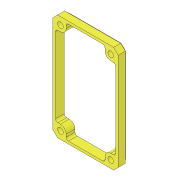
# Autodesk Inventor part: COXA_YAW_ROLL_ADPT_SPACER_2
Saved by Autodesk Inventor 2019.4 (Build 234330000, 330)
## iProperties
Created: 2019-11-06
Part Number: COXA_YAW_ROLL_ADPT_SPACER_2
Material: 一般
Document SubType Name: Modeling
Designer: y6tada
Density: 1 g/cm^3
Appearance: 滑らか - 黄
Author: y6tada
Autodesk Inventor part; units mm, degrees
ref_plane "YZ Plane" through (0, 0, 0) normal (1, 0, 0) x (0, 1, 0)
ref_plane "XZ Plane" through (0, 0, 0) normal (0, 1, 0) x (-1, 0, 0)
ref_plane "XY Plane" through (0, 0, 0) normal (0, 0, 1) x (1, 0, 0)
sketch "スケッチ1" plane through (0, 0, 0) normal (0, 0, 1) x (1, 0, 0)
  line L0 (-12.25, 11.25) -> (12.25, 11.25)
  line L1 (14.25, 9.25) -> (14.25, -33.25)
  line L2 (12.25, -35.25) -> (-12.25, -35.25)
  line L3 (-14.25, -33.25) -> (-14.25, 9.25)
  line L4 (-12.25, 11.25) -> (-14.25, 9.25)
  line L5 (12.25, 11.25) -> (14.25, 9.25)
  line L6 (14.25, -33.25) -> (12.25, -35.25)
  line L7 (-12.25, -35.25) -> (-14.25, -33.25)
  line L8 (0, 0) -> (-26.5626, 0) construction
  line L9 (0, 0) -> (0, 27.9433) construction
  line L10 (-11, 8) -> (11, 8) construction
  line L11 (11, 8) -> (11, -32) construction
  line L12 (11, -32) -> (-11, -32) construction
  line L13 (-11, -32) -> (-11, 8) construction
  line L14 (-13.15, -28.5) -> (-13.15, 4.5)
  line L15 (-7.5, 10.15) -> (7.5, 10.15)
  line L16 (13.15, 4.5) -> (13.15, -28.5)
  line L17 (7.5, -34.15) -> (-7.5, -34.15)
  line L18 (8.5, 8) -> (8.5, 9.15)
  line L19 (11, 5.5) -> (12.15, 5.5)
  arc A0 (8.5, 8) -> (11, 5.5) centre (11, 8) ccw
  line L20 (12.15, -29.5) -> (11, -29.5)
  line L21 (8.5, -32) -> (8.5, -33.15)
  arc A1 (11, -29.5) -> (8.5, -32) centre (11, -32) ccw
  line L22 (-8.5, 8) -> (-8.5, 9.15)
  line L23 (-11, 5.5) -> (-12.15, 5.5)
  arc A2 (-11, 5.5) -> (-8.5, 8) centre (-11, 8) ccw
  line L24 (-12.15, -29.5) -> (-11, -29.5)
  line L25 (-8.5, -32) -> (-8.5, -33.15)
  arc A3 (-8.5, -32) -> (-11, -29.5) centre (-11, -32) ccw
  arc A4 (8.5, 9.15) -> (7.5, 10.15) centre (7.5, 9.15) ccw
  arc A5 (13.15, 4.5) -> (12.15, 5.5) centre (12.15, 4.5) ccw
  arc A6 (12.15, -29.5) -> (13.15, -28.5) centre (12.15, -28.5) ccw
  arc A7 (7.5, -34.15) -> (8.5, -33.15) centre (7.5, -33.15) ccw
  arc A8 (-8.5, -33.15) -> (-7.5, -34.15) centre (-7.5, -33.15) ccw
  arc A9 (-13.15, -28.5) -> (-12.15, -29.5) centre (-12.15, -28.5) ccw
  arc A10 (-12.15, 5.5) -> (-13.15, 4.5) centre (-12.15, 4.5) ccw
  arc A11 (-7.5, 10.15) -> (-8.5, 9.15) centre (-7.5, 9.15) ccw
  point P0 (-14.25, 11.25)
  point P1 (14.25, -35.25)
  point P2 (14.25, 11.25)
  point P3 (-14.25, -35.25)
  point P4 (8.5, 10.15)
  point P5 (13.15, 5.5)
  point P6 (13.15, -29.5)
  point P7 (8.5, -34.15)
  point P8 (-8.5, 10.15)
  point P9 (-13.15, 5.5)
  point P10 (-13.15, -29.5)
  point P11 (-8.5, -34.15)
  dimension "d0" = 2
  dimension "d1" = 2
  dimension "d2" = 2
  dimension "d3" = 2
  dimension "d4" = 2
  dimension "d5" = 2
  dimension "d6" = 2
  dimension "d7" = 2
  dimension "d8" = 28.5
  dimension "d9" = 11.25
  dimension "d10" = 46.5
  dimension "d11" = 8
  dimension "d12" = 22
  dimension "d13" = 40
  dimension "d14" = 1.1
  dimension "d15" = 2.5
  dimension "d16" = 2.5
  dimension "d17" = 1.1
  dimension "d18" = 1.1
  dimension "d19" = 1
  constraints: 52 end point, 24 point on circle, 22 point on line, 20 tangent, 12 centre point, 10 symmetric about line, 7 coincident, 7 equal radius, 6 parallel, 6 perpendicular, 4 horizontal, 1 vertical, 5 other
  measures "d0" distance of L0.start point (-14.25, 11.25)
  measures "d1" distance of L3.end point (-14.25, 11.25)
  measures "d2" distance of L0.end point (14.25, 11.25)
  measures "d3" distance of L1.start point (14.25, 11.25)
  measures "d4" distance of L1.end point (14.25, -35.25)
  measures "d5" distance of L2.start point (14.25, -35.25)
  measures "d6" distance of L2.end point (-14.25, -35.25)
  measures "d7" distance of L3.start point (-14.25, -35.25)
  measures "d8" distance between parallel lines of L1 L3
  measures "d9" distance between parallel lines of L8 L0
  measures "d10" distance between parallel lines of L2 L0
  measures "d11" distance between parallel lines of L8 L10
  measures "d12" distance of L10.start L10.end
  measures "d13" distance of L12.end L10.start
  measures "d14" distance between parallel lines of L2 L17
  measures "d15" radius of A0
  measures "d16" radius of A1
  measures "d17" distance between parallel lines of L15 L0
  measures "d18" distance between parallel lines of L1 L16
  measures "d19" radius of A4
extrude "押し出し1" add sketch "スケッチ1" along normal blind 3.1
hole "穴1" at (-11, 8, 0) at (11, 8, 0) at (11, -32, 0) at (-11, -32, 0) direction (0, 0, 1) diameter 2.5 end through all
sketch "スケッチ3" plane through (0, 0, 0) normal (0, 0, -1) x (-1, 0, 0)
  line L0 (-12.25, 11.25) -> (12.25, 11.25) construction
  line L1 (12.25, 11.25) -> (14.25, 9.25) construction
  line L2 (14.25, 9.25) -> (14.25, -33.25) construction
  line L3 (14.25, -33.25) -> (12.25, -35.25) construction
  line L4 (12.25, -35.25) -> (-12.25, -35.25) construction
  line L5 (-12.25, -35.25) -> (-14.25, -33.25) construction
  line L6 (-14.25, -33.25) -> (-14.25, 9.25) construction
  line L7 (-14.25, 9.25) -> (-12.25, 11.25) construction
  line L8 (11.087, 10.625) -> (-11.087, 10.625)
  line L9 (-11.9911, 10.625) -> (-13.625, 8.9911) construction
  line L10 (-13.625, 8.087) -> (-13.625, -32.087)
  line L11 (-13.625, -32.9911) -> (-11.9911, -34.625) construction
  line L12 (-11.087, -34.625) -> (11.087, -34.625)
  line L13 (11.9911, -34.625) -> (13.625, -32.9911) construction
  line L14 (13.625, -32.087) -> (13.625, 8.087)
  line L15 (13.625, 8.9911) -> (11.9911, 10.625) construction
  line L16 (-13.1857, -33.1476) -> (-12.1476, -34.1857)
  line L17 (12.1476, -34.1857) -> (13.1857, -33.1476)
  line L18 (12.1476, 10.1857) -> (13.1857, 9.1476)
  line L19 (-13.1857, 9.1476) -> (-12.1476, 10.1857)
  arc A0 (-13.1857, 9.1476) -> (-13.625, 8.087) centre (-12.125, 8.087) ccw
  arc A1 (-11.087, 10.625) -> (-12.1476, 10.1857) centre (-11.087, 9.125) ccw
  arc A2 (12.1476, 10.1857) -> (11.087, 10.625) centre (11.087, 9.125) ccw
  arc A3 (13.625, 8.087) -> (13.1857, 9.1476) centre (12.125, 8.087) ccw
  arc A4 (13.1857, -33.1476) -> (13.625, -32.087) centre (12.125, -32.087) ccw
  arc A5 (11.087, -34.625) -> (12.1476, -34.1857) centre (11.087, -33.125) ccw
  arc A6 (-12.1476, -34.1857) -> (-11.087, -34.625) centre (-11.087, -33.125) ccw
  arc A7 (-13.625, -32.087) -> (-13.1857, -33.1476) centre (-12.125, -32.087) ccw
  arc A8 (-12.15, 5.5) -> (-13.15, 4.5) centre (-12.15, 4.5) ccw projected
  line L20 (-12.15, 5.5) -> (-11, 5.5) projected
  arc A9 (-11, 5.5) -> (-8.5, 8) centre (-11, 8) ccw projected
  line L21 (-8.5, 8) -> (-8.5, 9.15) projected
  arc A10 (-7.5, 10.15) -> (-8.5, 9.15) centre (-7.5, 9.15) ccw projected
  line L22 (-7.5, 10.15) -> (7.5, 10.15) projected
  arc A11 (8.5, 9.15) -> (7.5, 10.15) centre (7.5, 9.15) ccw projected
  line L23 (8.5, 9.15) -> (8.5, 8) projected
  arc A12 (8.5, 8) -> (11, 5.5) centre (11, 8) ccw projected
  line L24 (11, 5.5) -> (12.15, 5.5) projected
  arc A13 (13.15, 4.5) -> (12.15, 5.5) centre (12.15, 4.5) ccw projected
  circle A14 centre (11, 8) radius 1.25 projected
  line L25 (13.15, 4.5) -> (13.15, -28.5) projected
  arc A15 (12.15, -29.5) -> (13.15, -28.5) centre (12.15, -28.5) ccw projected
  line L26 (12.15, -29.5) -> (11, -29.5) projected
  arc A16 (11, -29.5) -> (8.5, -32) centre (11, -32) ccw projected
  line L27 (8.5, -32) -> (8.5, -33.15) projected
  arc A17 (7.5, -34.15) -> (8.5, -33.15) centre (7.5, -33.15) ccw projected
  circle A18 centre (11, -32) radius 1.25 projected
  line L28 (7.5, -34.15) -> (-7.5, -34.15) projected
  arc A19 (-8.5, -33.15) -> (-7.5, -34.15) centre (-7.5, -33.15) ccw projected
  line L29 (-8.5, -33.15) -> (-8.5, -32) projected
  arc A20 (-8.5, -32) -> (-11, -29.5) centre (-11, -32) ccw projected
  line L30 (-11, -29.5) -> (-12.15, -29.5) projected
  arc A21 (-13.15, -28.5) -> (-12.15, -29.5) centre (-12.15, -28.5) ccw projected
  circle A22 centre (-11, -32) radius 1.25 projected
  line L31 (-13.15, -28.5) -> (-13.15, 4.5) projected
  circle A23 centre (-11, 8) radius 1.25 projected
  point P0 (0, 0)
  dimension "d30" = 0.625
  dimension "d31" = 1.5
  dimension "d32" = 0.2
  constraints: 24 end point, 16 point on circle, 16 tangent, 8 centre point, 8 point on line, 7 equal radius, 4 parallel, 3 equal length, 7 other
  measures "d30" distance between parallel lines of L0 L8
  measures "d31" radius of A0
  measures "d32" distance between parallel lines of L16 L11
extrude "押し出し2" add sketch "スケッチ3" along normal blind 0.75
equation "\"d1\" = d0"
equation "\"d2\" = d0"
equation "\"d3\" = d2"
equation "\"d4\" = d0"
equation "\"d5\" = d4"
equation "\"d6\" = d0"
equation "\"d7\" = d6"
